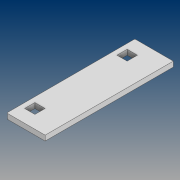
# Autodesk Inventor part: 15_Top_truc_vit
Saved by Autodesk Inventor 2021 (Build 250183000, 183)
## iProperties
Created: 2024-04-04
Part Number: 15_Top_truc_vit
Material: Generic
Document SubType Name: Modeling
Designer: Admin
Density: 1 g/cm^3
Appearance: Default
Author: Admin
Autodesk Inventor part; units mm, degrees
ref_plane "YZ Plane" through (0, 0, 0) normal (1, 0, 0) x (0, 1, 0)
ref_plane "XZ Plane" through (0, 0, 0) normal (0, 1, 0) x (-1, 0, 0)
ref_plane "XY Plane" through (0, 0, 0) normal (0, 0, 1) x (1, 0, 0)
sketch "Sketch1" plane through (0, 0, 0) normal (0, 1, 0) x (-1, 0, 0)
  line L0 (-20, 125) -> (-20, -125)
  line L1 (-20, -125) -> (20, -125)
  line L2 (20, -125) -> (20, 125)
  line L3 (20, 125) -> (-20, 125)
  line L4 (-20, 125) -> (20, -125) construction
  line L5 (-20, -125) -> (20, 125) construction
  line L6 (0, 90) -> (0, -90) construction
  line L7 (20, 0) -> (-20, 0) construction
  line L8 (-10, 100) -> (10, 100)
  line L9 (10, 100) -> (10, 80)
  line L10 (10, 80) -> (-10, 80)
  line L11 (-10, 80) -> (-10, 100)
  line L12 (-10, 100) -> (10, 80) construction
  line L13 (10, 100) -> (-10, 80) construction
  line L14 (-10, -80) -> (10, -80)
  line L15 (10, -80) -> (10, -100)
  line L16 (10, -100) -> (-10, -100)
  line L17 (-10, -100) -> (-10, -80)
  line L18 (-10, -80) -> (10, -100) construction
  line L19 (10, -80) -> (-10, -100) construction
  line L20 (-20, 125) -> (-20, -125)
  line L21 (-20, -125) -> (-55, -125)
  line L22 (-55, -125) -> (-55, 125)
  line L23 (-55, 125) -> (-20, 125)
  point P0 (0, 0)
  point P1 (0, 0)
  dimension "d0" = 250
  dimension "d1" = 40
  dimension "d2" = 180
  dimension "d3" = 20
  dimension "d4" = 35
  constraints: 48 end point, 10 midpoint, 8 parallel, 4 perpendicular, 3 horizontal, 2 equal length, 2 vertical, 1 point on line, 1 symmetric about line
  measures "d0" distance of L1.end L2.end
  measures "d1" distance between parallel lines of L0 L2
  measures "d2" distance of L6.start L6.end
  measures "d3" distance of L15.end L16.end
  measures "d4" distance between parallel lines of L0 L22
extrude "Extrusion1" add sketch "Sketch1" along normal mid plane 10
fillet "Fillet1" radius 2 2 edges at (-20, 0, 125) (-20, 0, -125)
body "Solid1"
